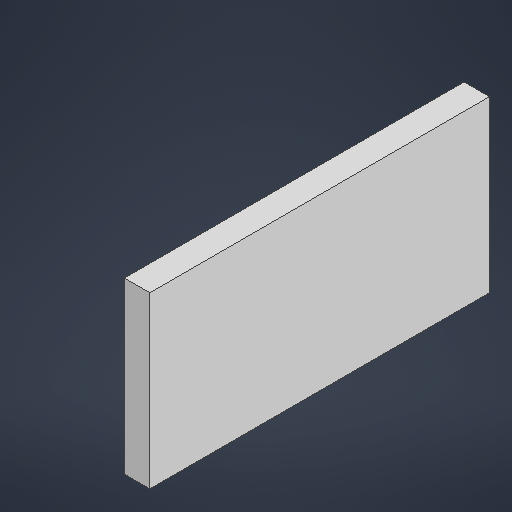
# Autodesk Inventor part: Part9
Saved by Autodesk Inventor 2026 (Build 300175000, 175)
## iProperties
Created: 2025-04-11
Part Number: Part9
Material: Generic
Document SubType Name: Modeling
Designer: janpa
Density: 1 g/cm^3
Appearance: Default
Author: janpa
Autodesk Inventor part; units mm, degrees
ref_plane "YZ Plane" through (0, 0, 0) normal (1, 0, 0) x (0, 1, 0)
ref_plane "XZ Plane" through (0, 0, 0) normal (0, 1, 0) x (-1, 0, 0)
ref_plane "XY Plane" through (0, 0, 0) normal (0, 0, 1) x (1, 0, 0)
sketch "Sketch1" plane through (0, 0, 0) normal (0, 1, 0) x (-1, 0, 0)
  line L0 (4.0517, 5) -> (-7.9483, 5)
  line L1 (-7.9483, 5) -> (-7.9483, -5)
  line L2 (-7.9483, -5) -> (4.0517, -5)
  line L3 (4.0517, -5) -> (4.0517, 5)
  circle A0 centre (0, 0) radius 2.85
  dimension "d0" = 5.7
  dimension "d1" = 10
  dimension "d2" = 5
  dimension "d3" = 12
  constraints: 8 end point, 2 parallel, 1 centre point, 1 coincident, 1 horizontal, 1 perpendicular
  measures "d0" diameter of A0
  measures "d1" distance of L2.end L0.start
  measures "d2" distance from line of L0 A0.centre
  measures "d3" distance of L0.start L0.end
extrude "Extrusion1" add sketch "Sketch1" along normal blind 3
sketch "Sketch2" plane through (7.9483, 0, 5) normal (1, 0, 0) x (0, 0, -1)
  line L0 (-15, 0) -> (25, 0)
  line L1 (25, 0) -> (25, 20)
  line L2 (25, 20) -> (-15, 20)
  line L3 (-15, 20) -> (-15, 0)
  line L4 (0, 0) -> (0, 3) projected
  line L5 (10, 0) -> (0, 0) projected
  point P0 (5, 0)
  dimension "d6" = 40
  dimension "d7" = 20
  dimension "d8" = 15
  constraints: 8 end point, 2 parallel, 1 collinear, 1 horizontal, 1 perpendicular
  measures "d6" distance of L2.end L1.end
  measures "d7" distance of L1.end L0.end
  measures "d8" distance between parallel lines of L3 L4
extrude "Extrusion2" add sketch "Sketch2" along normal blind 3
body "Solid1"
